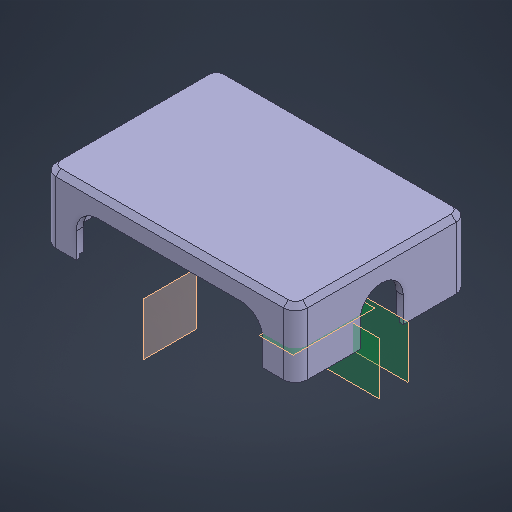
# Autodesk Inventor part: case2
Saved by Autodesk Inventor 2025.2 (Build 292293000, 293)
## iProperties
Created: 2025-10-05
Part Number: case2
Material: Generic
Document SubType Name: Modeling
Designer: micyg
Density: 1 g/cm^3
Appearance: Default
Sheet Metal Rule: Default
Author: micyg
## iProperties of the stored document case2_3DPrint.ipt
Created: 2025-10-05
Part Number: case2_3DPrint
Material: Generic
Document SubType Name: Modeling
Designer: micyg
Density: 1 g/cm^3
Appearance: Default
Author: micyg
Autodesk Inventor part; units mm, degrees
ref_plane "YZ Plane" through (0, 0, 0) normal (1, 0, 0) x (0, 1, 0)
ref_plane "XZ Plane" through (0, 0, 0) normal (0, 1, 0) x (-1, 0, 0)
ref_plane "XY Plane" through (0, 0, 0) normal (0, 0, 1) x (1, 0, 0)
sketch "Sketch1" plane through (0, 0, 0) normal (0, 1, 0) x (-1, 0, 0)
  line L0 (0, 0) -> (105.2, 0)
  line L1 (105.2, 0) -> (105.2, -72.2)
  line L2 (105.2, -72.2) -> (0, -72.2)
  line L3 (0, -72.2) -> (0, 0)
  dimension "d0" = 105.2
  dimension "d1" = 72.2
  constraints: 8 end point, 2 parallel, 1 horizontal, 1 perpendicular
  measures "d0" distance of L1.end L2.end
  measures "d1" distance of L0.end L1.end
extrude "Extrusion1" add sketch "Sketch1" along normal blind 28
fillet "Fillet1" radius 5 4 edges at (-105.2, 14, 0) (0, 14, 0) (-105.2, 14, -72.2) (0, 14, -72.2)
chamfer "Chamfer1" distance 2 angle 45 8 edges at (-52.6, 28, 0) (-1.4645, 28, -1.4645) (0, 28, -36.1) (-1.4645, 28, -70.7355) (-52.6, 28, -72.2) (-103.7355, 28, -70.7355) (-105.2, 28, -36.1) (-103.7355, 28, -1.4645)
shell "Shell2" thickness 3 removed faces 1 at (-36.7333, 0, -24.0667)
sketch "Sketch2" plane through (0, 0, 0) normal (0, -1, 0) x (1, 0, 0)
  arc A0 (-5, -69.2) -> (-3, -67.2) centre (-5, -67.2) ccw projected
  line L0 (-5, -69.2) -> (-100.2, -69.2) projected
  arc A1 (-102.2, -67.2) -> (-100.2, -69.2) centre (-100.2, -67.2) ccw projected
  line L1 (-102.2, -67.2) -> (-102.2, -5) projected
  arc A2 (-100.2, -3) -> (-102.2, -5) centre (-100.2, -5) ccw projected
  line L2 (-100.2, -3) -> (-5, -3) projected
  arc A3 (-3, -5) -> (-5, -3) centre (-5, -5) ccw projected
  line L3 (-3, -5) -> (-3, -67.2) projected
  arc A4 (-5, -72.2) -> (0, -67.2) centre (-5, -67.2) ccw projected
  line L4 (0, -5) -> (0, -67.2) projected
  arc A5 (0, -5) -> (-5, 0) centre (-5, -5) ccw projected
  line L5 (-100.2, 0) -> (-5, 0) projected
  arc A6 (-100.2, 0) -> (-105.2, -5) centre (-100.2, -5) ccw projected
  line L6 (-105.2, -67.2) -> (-105.2, -5) projected
  arc A7 (-105.2, -67.2) -> (-100.2, -72.2) centre (-100.2, -67.2) ccw projected
  line L7 (-5, -72.2) -> (-100.2, -72.2) projected
  arc A8 (-5, -70.8) -> (-1.4, -67.2) centre (-5, -67.2) ccw
  line L8 (-5, -70.8) -> (-100.2, -70.8)
  arc A9 (-103.8, -67.2) -> (-100.2, -70.8) centre (-100.2, -67.2) ccw
  line L9 (-103.8, -67.2) -> (-103.8, -5)
  arc A10 (-100.2, -1.4) -> (-103.8, -5) centre (-100.2, -5) ccw
  line L10 (-100.2, -1.4) -> (-5, -1.4)
  arc A11 (-1.4, -5) -> (-5, -1.4) centre (-5, -5) ccw
  line L11 (-1.4, -5) -> (-1.4, -67.2)
  point P0 (0, 0)
  dimension "d8" = 1.4
  constraints: 8 end point, 8 point on circle, 4 centre point, 7 other
  measures "d8" distance between parallel lines of L4 L11
extrude "Extrusion2" cut sketch "Sketch2" against normal blind 1.6 contours L8 A9 L9 A10 L10 A11 L11 A8
ref_plane "Work Plane2" through (-52.6, 0, 0) normal (1, 0, 0) x (0, 1, 0)
ref_plane "Work Plane3" through (0, 0, -36.1) normal (0, 0, -1) x (-1, 0, 0)
ref_plane "Work Plane4" through (0, 12.5, 0) normal (0, -1, 0) x (1, 0, 0)
sketch "Sketch19" plane through (-52.6, 0, 0) normal (1, 0, 0) x (0, 1, 0)
  line L0 (1.6, -3) -> (24.7574, -3) projected
  line L1 (24.7574, -3) -> (1.6, -3) projected
  arc A0 (25, -4) -> (24, -3) centre (24, -4) ccw projected
  arc A1 (25, -4) -> (24, -3) centre (24, -4) ccw projected
  line L2 (25, -68.2) -> (25, -67.2) projected
  line L3 (25, -67.2) -> (25, -5) projected
  line L4 (25, -5) -> (25, -4) projected
  line L5 (25, -4) -> (25, -5) projected
  line L6 (25, -5) -> (25, -67.2) projected
  line L7 (25, -67.2) -> (25, -68.2) projected
  line L8 (25, -5.7) -> (18, -5.7)
  line L9 (17, -5.7) -> (18, -6.7) construction
  line L10 (18, -6.7) -> (18, -5.7)
  line L11 (18, -5.7) -> (17, -5.7) construction
  line L12 (18, -6.7) -> (25, -13.7)
  line L13 (0, -67.2) -> (0, -70.8) projected
  line L14 (0, -70.8) -> (0, -67.2) projected
  line L15 (0, -67.2) -> (0, -5) projected
  line L16 (0, -5) -> (0, -1.4) projected
  line L17 (0, -1.4) -> (0, -5) projected
  line L18 (0, -5) -> (0, -67.2) projected
  line L19 (0, -67.2) -> (0, -72.2) projected
  line L20 (0, -5) -> (0, -67.2) projected
  line L21 (0, 0) -> (0, -5) projected
  line L22 (0, -5) -> (0, 0) projected
  line L23 (0, -67.2) -> (0, -5) projected
  line L24 (0, -72.2) -> (0, -67.2) projected
  dimension "d103" = 45
  dimension "d104" = 2.7
  dimension "d105" = 1
  dimension "d106" = 18
  constraints: 10 end point, 4 perpendicular, 2 point on line, 1 collinear
  measures "d103" angle of L3 L9
  measures "d104" distance between parallel lines of L0 L8
  measures "d105" distance from line of L9.end L8
  measures "d106" distance between parallel lines of L15 L10
extrude "Extrusion15" add sketch "Sketch19" against normal up to surface (49.6 mm away)
mirror "Mirror9" about plane through (-52.6, 0, 0) normal (1, 0, 0) of "Extrusion15"
mirror "Mirror10" about plane through (0, 0, -36.1) normal (0, 0, -1) of "Extrusion15", "Mirror9"
sketch "Sketch9" plane through (0, 12.5, 0) normal (0, -1, 0) x (1, 0, 0)
  arc A0 (-5, -70.8) -> (-1.4, -67.2) centre (-5, -67.2) ccw projected
  line L0 (-5, -70.8) -> (-100.2, -70.8) projected
  arc A1 (-103.8, -67.2) -> (-100.2, -70.8) centre (-100.2, -67.2) ccw projected
  line L1 (-103.8, -67.2) -> (-103.8, -5) projected
  arc A2 (-100.2, -1.4) -> (-103.8, -5) centre (-100.2, -5) ccw projected
  line L2 (-100.2, -1.4) -> (-5, -1.4) projected
  arc A3 (-1.4, -5) -> (-5, -1.4) centre (-5, -5) ccw projected
  line L3 (-1.4, -5) -> (-1.4, -67.2) projected
  arc A4 (-5, -72.2) -> (0, -67.2) centre (-5, -67.2) ccw projected
  line L4 (0, -5) -> (0, -67.2) projected
  arc A5 (0, -5) -> (-5, 0) centre (-5, -5) ccw projected
  line L5 (-100.2, 0) -> (-5, 0) projected
  arc A6 (-100.2, 0) -> (-105.2, -5) centre (-100.2, -5) ccw projected
  line L6 (-105.2, -67.2) -> (-105.2, -5) projected
  arc A7 (-105.2, -67.2) -> (-100.2, -72.2) centre (-100.2, -67.2) ccw projected
  line L7 (-5, -72.2) -> (-100.2, -72.2) projected
  line L8 (-5, -70.8) -> (-100.2, -70.8) projected
  arc A8 (-5, -70.8) -> (-1.4, -67.2) centre (-5, -67.2) ccw projected
  line L9 (-1.4, -5) -> (-1.4, -67.2) projected
  arc A9 (-1.4, -5) -> (-5, -1.4) centre (-5, -5) ccw projected
  line L10 (-100.2, -1.4) -> (-5, -1.4) projected
  arc A10 (-100.2, -1.4) -> (-103.8, -5) centre (-100.2, -5) ccw projected
  line L11 (-103.8, -67.2) -> (-103.8, -5) projected
  arc A11 (-103.8, -67.2) -> (-100.2, -70.8) centre (-100.2, -67.2) ccw projected
  line L12 (-102.2, -5) -> (-102.2, -67.2) projected
  arc A12 (-100.2, -3) -> (-102.2, -5) centre (-100.2, -5) ccw projected
  line L13 (-5, -3) -> (-100.2, -3) projected
  arc A13 (-3, -5) -> (-5, -3) centre (-5, -5) ccw projected
  line L14 (-3, -67.2) -> (-3, -5) projected
  arc A14 (-5, -69.2) -> (-3, -67.2) centre (-5, -67.2) ccw projected
  line L15 (-100.2, -69.2) -> (-5, -69.2) projected
  arc A15 (-102.2, -67.2) -> (-100.2, -69.2) centre (-100.2, -67.2) ccw projected
  line L16 (-96.7, -8.6) -> (-8.7, -8.6) construction
  line L17 (-8.7, -8.6) -> (-8.7, -63.6) construction
  line L18 (-8.7, -63.6) -> (-96.7, -63.6) construction
  line L19 (-96.7, -63.6) -> (-96.7, -8.6) construction
  circle A16 centre (-96.7, -8.6) radius 1.5
  circle A17 centre (-8.7, -8.6) radius 1.5
  circle A18 centre (-96.7, -63.6) radius 1.5
  circle A19 centre (-8.7, -63.6) radius 1.5
  line L20 (-52.7, -8.6) -> (-52.7, -63.6) construction
  line L21 (-101.7, -3.6) -> (-3.7, -3.6) construction
  line L22 (-3.7, -3.6) -> (-3.7, -68.6) construction
  line L23 (-3.7, -68.6) -> (-101.7, -68.6) construction
  line L24 (-101.7, -68.6) -> (-101.7, -3.6) construction
  line L25 (-101.7, -36.1) -> (-3.7, -36.1) construction
  line L26 (-52.6, 0) -> (-52.6, -72.2) construction
  line L27 (-105.2, -36.1) -> (0, -36.1) construction
  line L28 (-93.2, -3) -> (-93.2, -8.6)
  line L29 (-102.2, -12.1) -> (-102.2, -5)
  arc A20 (-96.7, -12.1) -> (-93.2, -8.6) centre (-96.7, -8.6) ccw
  line L30 (-96.7, -12.1) -> (-102.2, -12.1)
  line L31 (-100.2, -3) -> (-93.2, -3)
  line L32 (-93.2, -69.2) -> (-93.2, -63.6)
  arc A21 (-93.2, -63.6) -> (-96.7, -60.1) centre (-96.7, -63.6) ccw
  line L33 (-96.7, -60.1) -> (-102.2, -60.1)
  arc A22 (-12.2, -8.6) -> (-8.7, -12.1) centre (-8.7, -8.6) ccw
  line L34 (-3, -12.1) -> (-3, -5)
  line L35 (-12.2, -3) -> (-12.2, -8.6)
  line L36 (-8.7, -12.1) -> (-3, -12.1)
  line L37 (-5, -3) -> (-12.2, -3)
  arc A23 (-8.7, -60.1) -> (-12.2, -63.6) centre (-8.7, -63.6) ccw
  line L38 (-12.2, -69.2) -> (-12.2, -63.6)
  line L39 (-8.7, -60.1) -> (-3, -60.1)
  line L40 (-93.2, -3) -> (-95.2, -3)
  line L41 (-95.2, -3) -> (-95.2, -6)
  line L42 (-95.2, -6) -> (-93.2, -6)
  line L43 (-93.2, -6) -> (-93.2, -3)
  line L44 (-12.2, -3) -> (-10.2, -3)
  line L45 (-10.2, -3) -> (-10.2, -6)
  line L46 (-10.2, -6) -> (-12.2, -6)
  line L47 (-12.2, -6) -> (-12.2, -3)
  line L48 (-95.2, -69.2) -> (-95.2, -66.2)
  line L49 (-95.2, -66.2) -> (-93.2, -66.2)
  line L50 (-10.2, -69.2) -> (-10.2, -66.2)
  line L51 (-10.2, -66.2) -> (-12.2, -66.2)
  arc A24 (-3, -5) -> (-5, -3) centre (-5, -5) ccw projected
  line L52 (-5, -3) -> (-100.2, -3) projected
  arc A25 (-100.2, -3) -> (-102.2, -5) centre (-100.2, -5) ccw projected
  line L53 (-102.2, -5) -> (-102.2, -67.2) projected
  arc A26 (-102.2, -67.2) -> (-100.2, -69.2) centre (-100.2, -67.2) ccw projected
  line L54 (-100.2, -69.2) -> (-5, -69.2) projected
  arc A27 (-5, -69.2) -> (-3, -67.2) centre (-5, -67.2) ccw projected
  line L55 (-3, -67.2) -> (-3, -5) projected
  arc A28 (0, -5) -> (-5, 0) centre (-5, -5) ccw projected
  line L56 (0, -5) -> (0, -67.2) projected
  arc A29 (-5, -72.2) -> (0, -67.2) centre (-5, -67.2) ccw projected
  line L57 (-5, -72.2) -> (-100.2, -72.2) projected
  arc A30 (-105.2, -67.2) -> (-100.2, -72.2) centre (-100.2, -67.2) ccw projected
  line L58 (-105.2, -67.2) -> (-105.2, -5) projected
  arc A31 (-100.2, 0) -> (-105.2, -5) centre (-100.2, -5) ccw projected
  line L59 (-100.2, 0) -> (-5, 0) projected
  arc A32 (-3, -5) -> (-5, -3) centre (-5, -5) ccw projected
  line L60 (-5, -3) -> (-100.2, -3) projected
  arc A33 (-100.2, -3) -> (-102.2, -5) centre (-100.2, -5) ccw projected
  line L61 (-102.2, -5) -> (-102.2, -67.2) projected
  arc A34 (-102.2, -67.2) -> (-100.2, -69.2) centre (-100.2, -67.2) ccw projected
  line L62 (-100.2, -69.2) -> (-5, -69.2) projected
  arc A35 (-5, -69.2) -> (-3, -67.2) centre (-5, -67.2) ccw projected
  line L63 (-3, -67.2) -> (-3, -5) projected
  arc A36 (0, -5) -> (-5, 0) centre (-5, -5) ccw projected
  line L64 (0, -5) -> (0, -67.2) projected
  arc A37 (-5, -72.2) -> (0, -67.2) centre (-5, -67.2) ccw projected
  line L65 (-5, -72.2) -> (-100.2, -72.2) projected
  arc A38 (-105.2, -67.2) -> (-100.2, -72.2) centre (-100.2, -67.2) ccw projected
  line L66 (-105.2, -67.2) -> (-105.2, -5) projected
  arc A39 (-100.2, 0) -> (-105.2, -5) centre (-100.2, -5) ccw projected
  line L67 (-100.2, 0) -> (-5, 0) projected
  point P0 (-52.7, -36.1)
  dimension "d137" = 88
  dimension "d138" = 55
  dimension "d139" = 3
  dimension "d140" = 3
  dimension "d141" = 3
  dimension "d142" = 3
  dimension "d143" = 98
  dimension "d144" = 65
  dimension "d145" = 0.5
  dimension "d147" = 2
  dimension "d148" = 2
  dimension "d149" = 3
  dimension "d150" = 2
  constraints: 72 end point, 16 symmetric about line, 12 parallel, 12 point on circle, 10 midpoint, 8 centre point, 6 horizontal, 6 perpendicular, 6 point on line, 5 coincident, 4 tangent, 1 collinear, 3 other
  measures "d137" distance of L16.start L16.end
  measures "d138" distance of L18.end L16.start
  measures "d139" diameter of A16
  measures "d140" diameter of A19
  measures "d141" diameter of A17
  measures "d142" diameter of A18
  measures "d143" distance of L21.start L21.end
  measures "d144" distance of L23.end L21.start
  measures "d145" distance between parallel lines of L12 L24
  measures "d147" radial gap between concentric circles of A16 A20
  measures "d148" radial gap between concentric circles of A22 A17
  measures "d149" distance between parallel lines of L13 L42
  measures "d150" distance between parallel lines of L28 L41
extrude "Extrusion13" add sketch "Sketch9" against normal up to surface (12.5 mm away) contours A12 L13 L41 L42 L28 A20 L30 L12 | L33 A21 L32 L49 L48 L15 A15 L12 | L13 A13 L14 L36 A22 L35 L46 L45 | L50 L51 L38 A23 L39 L14 A14 L15 | A16 | A17 | A18 | A19
sketch "Sketch18" plane through (-105.2, 0, -67.2) normal (-1, 0, 0) x (0, 0, 1)
  line L0 (26.03, 2.015) -> (26.03, 2.615)
  arc A0 (27.81, 4.395) -> (26.03, 2.615) centre (27.81, 2.615) ccw
  arc A1 (26.03, 2.015) -> (27.81, 0.235) centre (27.81, 2.015) ccw construction
  line L1 (27.81, 0.235) -> (31.1061, 0.235)
  line L2 (34.19, 0.235) -> (31.1061, 0.235)
  arc A2 (34.19, 0.235) -> (35.97, 2.015) centre (34.19, 2.015) ccw construction
  line L3 (35.97, 2.615) -> (35.97, 2.015)
  arc A3 (35.97, 2.615) -> (34.19, 4.395) centre (34.19, 2.615) ccw
  line L4 (27.81, 4.395) -> (34.19, 4.395)
  line L5 (35.97, 2.015) -> (26.03, 2.015) construction
  line L6 (26.03, 2.015) -> (26.03, 0.235)
  line L7 (35.97, 0.235) -> (35.97, 2.015)
  line L8 (31, 0.935) -> (31, 0.735) projected
  line L9 (27.81, 0.935) -> (31, 0.935) projected
  arc A4 (26.73, 2.015) -> (27.81, 0.935) centre (27.81, 2.015) ccw projected
  line L10 (26.73, 2.615) -> (26.73, 2.015) projected
  arc A5 (27.81, 3.695) -> (26.73, 2.615) centre (27.81, 2.615) ccw projected
  line L11 (31, 3.695) -> (27.81, 3.695) projected
  line L12 (31, 3.895) -> (31, 3.695) projected
  line L13 (31, 3.895) -> (27.81, 3.895) projected
  arc A6 (27.81, 3.895) -> (26.53, 2.615) centre (27.81, 2.615) ccw projected
  line L14 (26.53, 2.615) -> (26.53, 2.015) projected
  arc A7 (26.53, 2.015) -> (27.81, 0.735) centre (27.81, 2.015) ccw projected
  line L15 (27.81, 0.735) -> (31, 0.735) projected
  line L16 (31, 0.935) -> (31, 0.735) projected
  line L17 (34.19, 0.735) -> (31, 0.735) projected
  arc A8 (34.19, 0.735) -> (35.47, 2.015) centre (34.19, 2.015) ccw projected
  line L18 (35.47, 2.615) -> (35.47, 2.015) projected
  arc A9 (35.47, 2.615) -> (34.19, 3.895) centre (34.19, 2.615) ccw projected
  line L19 (31, 3.895) -> (34.19, 3.895) projected
  line L20 (31, 3.895) -> (31, 3.695) projected
  line L21 (31, 3.695) -> (34.19, 3.695) projected
  arc A10 (35.27, 2.615) -> (34.19, 3.695) centre (34.19, 2.615) ccw projected
  line L22 (35.27, 2.615) -> (35.27, 2.015) projected
  arc A11 (34.19, 0.935) -> (35.27, 2.015) centre (34.19, 2.015) ccw projected
  line L23 (34.19, 0.935) -> (31, 0.935) projected
  line L24 (26.03, 0.235) -> (35.97, 0.235)
  line L25 (0, 0) -> (0, 26) projected
  line L26 (0, 0) -> (62.2, 0) projected
  line L27 (62.2, 26) -> (62.2, 0) projected
  line L28 (0, 0) -> (62.2, 0) projected
  line L29 (35.97, 0.235) -> (26.03, 0.235)
  line L30 (26.03, 0.235) -> (26.03, 0)
  line L31 (26.03, 0) -> (35.97, 0)
  line L32 (35.97, 0) -> (35.97, 0.235)
  line L33 (0, 26) -> (62.2, 26) projected
  point P0 (67.2, 0)
  dimension "d136" = 0.5
  constraints: 26 end point, 8 point on circle, 8 tangent, 4 centre point, 4 coincident, 4 horizontal, 3 parallel, 2 perpendicular, 2 point on line, 1 collinear
  measures "d136" distance between parallel lines of L4 L13
extrude "Extrusion14" cut sketch "Sketch18" against normal up to surface (3 mm away) contours L0 A0 L4 A3 L3 L7 L24 L2 L1 L6 | L24 L1 L2 L32 L26 L30 | L23 A11 L22 A10 L21 L12 L19 A9 L18 A8 L17 L8 | L8 L15 A7 L14 A6 L13 L12 L11 A5 L10 A4 L9 | L9 A4 L10 A5 L11 L21 A10 L22 A11 L23
sketch "Sketch20" plane through (0, 0, -5) normal (1, 0, 0) x (0, 0, -1)
  circle A0 centre (31.1, 10.585) radius 9
  line L0 (40.1, 10.585) -> (22.1, 10.585) construction
  line L1 (22.1, 10.585) -> (22.1, 0)
  line L2 (22.1, 0) -> (40.1, 0)
  line L3 (40.1, 0) -> (40.1, 10.585)
  line L4 (0, 0) -> (0, 26) construction
  line L5 (0, 0) -> (62.2, 0) construction
  line L6 (62.2, 26) -> (62.2, 0) construction
  line L7 (0, 0) -> (62.2, 0) construction
  circle A1 centre (31.1, 10.585) radius 7 construction
  line L8 (0, 26) -> (62.2, 26) projected
  point P0 (-5, 0)
  dimension "d109" = 18
  constraints: 8 end point, 2 parallel, 2 point on circle, 1 centre point, 1 coincident, 1 horizontal, 1 midpoint, 1 perpendicular, 1 point on line, 1 tangent
  measures "d109" diameter of A0
extrude "Extrusion16" cut sketch "Sketch20" against normal up to surface (3 mm away)
sketch "Sketch21" plane through (-5, 0, -72.2) normal (0, 0, -1) x (-1, 0, 0)
  line L0 (87.5, 0.585) -> (67.5, 0.585) construction
  line L1 (87.5, 0.585) -> (87.5, 20.085) construction
  line L2 (67.5, 20.085) -> (87.5, 20.085) construction
  line L3 (67.5, 20.085) -> (67.5, 0.585) construction
  line L4 (67.5, 0.585) -> (47.5, 0.585) construction
  line L5 (67.5, 0.585) -> (67.5, 20.085) construction
  line L6 (47.5, 20.085) -> (67.5, 20.085) construction
  line L7 (47.5, 20.085) -> (47.5, 0.585) construction
  line L8 (47.5, 0.585) -> (27.5, 0.585) construction
  line L9 (47.5, 0.585) -> (47.5, 20.085) construction
  line L10 (27.5, 20.085) -> (47.5, 20.085) construction
  line L11 (27.5, 20.085) -> (27.5, 0.585) construction
  line L12 (27.5, 0.585) -> (7.5, 0.585) construction
  line L13 (27.5, 0.585) -> (27.5, 20.085) construction
  line L14 (7.5, 20.085) -> (27.5, 20.085) construction
  line L15 (7.5, 20.085) -> (7.5, 0.585) construction
  circle A0 centre (17.7, 10.585) radius 9
  circle A1 centre (37.7, 10.585) radius 9
  circle A2 centre (57.7, 10.585) radius 9
  circle A3 centre (77.7, 10.585) radius 9
  line L16 (0, 0) -> (0, 26) construction
  line L17 (0, 0) -> (95.2, 0) projected
  line L18 (95.2, 26) -> (95.2, 0) construction
  line L19 (8.7, 10.585) -> (26.7, 10.585) construction
  line L20 (26.7, 10.585) -> (26.7, 0)
  line L21 (26.7, 0) -> (8.7, 0)
  line L22 (8.7, 0) -> (8.7, 10.585)
  line L23 (28.7, 10.585) -> (46.7, 10.585) construction
  line L24 (46.7, 10.585) -> (46.7, 0)
  line L25 (46.7, 0) -> (28.7, 0)
  line L26 (28.7, 0) -> (28.7, 10.585)
  line L27 (48.7, 10.585) -> (66.7, 10.585) construction
  line L28 (66.7, 10.585) -> (66.7, 0)
  line L29 (66.7, 0) -> (48.7, 0)
  line L30 (48.7, 0) -> (48.7, 10.585)
  line L31 (68.7, 10.585) -> (86.7, 10.585) construction
  line L32 (86.7, 10.585) -> (86.7, 0)
  line L33 (86.7, 0) -> (68.7, 0)
  line L34 (68.7, 0) -> (68.7, 10.585)
  line L35 (17.7, 19.585) -> (77.7, 19.585)
  circle A4 centre (17.7, 10.585) radius 7 projected
  circle A5 centre (37.7, 10.585) radius 7 projected
  circle A6 centre (57.7, 10.585) radius 7 projected
  circle A7 centre (77.7, 10.585) radius 7 projected
  line L36 (0, 26) -> (95.2, 26) projected
  point P0 (8.7, 0)
  dimension "d132" = 18
  dimension "d133" = 18
  dimension "d134" = 18
  dimension "d135" = 18
  constraints: 34 end point, 10 point on circle, 8 parallel, 6 point on line, 4 centre point, 4 horizontal, 4 perpendicular, 4 tangent, 3 coincident, 3 midpoint, 2 concentric
  measures "d132" diameter of A0
  measures "d133" diameter of A1
  measures "d134" diameter of A2
  measures "d135" diameter of A3
extrude "Extrusion17" cut sketch "Sketch21" against normal up to surface (3 mm away) contours A0 | L20 L17 L22 A0 | A0 L35 A1 L26 L17 L20 | L35 A2 L30 L17 L24 A1 | A1 | L26 A1 L24 L17 | L35 A3 L34 L17 L28 A2 | A2 | L28 L17 L30 A2 | A3 | L32 L17 L34 A3 | A4 | A5 | A6 | A7
mirror "Mirror11" about plane through (0, 0, -36.1) normal (0, 0, -1) of "Extrusion17"
ref_plane "Work Plane6" through (0, 0, -24.1) normal (0, 0, -1) x (-1, 0, 0)
sketch "Sketch22" plane through (0, 0, -24.1) normal (0, 0, -1) x (-1, 0, 0)
  line L0 (3, 10.585) -> (3, 1.6) projected
  line L1 (3, 1.6) -> (3, 12.5) projected
  line L2 (3, 12.5) -> (3, 1.6) projected
  line L3 (3, 1.6) -> (3, 10.585) projected
  line L4 (3, 10.585) -> (3, 10.585) projected
  arc A0 (4, 25) -> (3, 24) centre (4, 24) ccw projected
  arc A1 (4, 25) -> (3, 24) centre (4, 24) ccw projected
  line L5 (101.9574, 25) -> (3.2426, 25) projected
  line L6 (3.2426, 25) -> (101.9574, 25) projected
  arc A2 (102.2, 24) -> (101.2, 25) centre (101.2, 24) ccw projected
  arc A3 (102.2, 24) -> (101.2, 25) centre (101.2, 24) ccw projected
  line L7 (102.2, 2.615) -> (102.2, 1.6) projected
  line L8 (102.2, 1.6) -> (102.2, 12.5) projected
  line L9 (102.2, 12.5) -> (102.2, 1.6) projected
  line L10 (102.2, 1.6) -> (102.2, 2.615) projected
  line L11 (102.2, 2.615) -> (102.2, 4.395) projected
  line L12 (102.2, 4.395) -> (102.2, 2.615) projected
  line L13 (3, 5) -> (23, 25)
  line L14 (82.2, 25) -> (102.2, 5)
  line L15 (101.2, 25) -> (10.2, 25) projected
  line L16 (12.115, 25) -> (6.7, 19.585)
  line L17 (6.7, 19.585) -> (5.7, 19.585)
  line L18 (5.7, 19.585) -> (5.7, 25)
  line L19 (100.2, 0) -> (91.7, 0) projected
  line L20 (5, 26) -> (5, 0) projected
  line L21 (100.2, 0) -> (100.2, 26) projected
  line L22 (102.2, 23.4) -> (102.2, 24.7574) projected
  line L23 (3, 24.7574) -> (3, 23.4) projected
  line L24 (102.2, 24.7574) -> (102.2, 23.4) projected
  line L25 (3, 23.4) -> (3, 24.7574) projected
  line L26 (91.7, 0) -> (91.7, 10.585) construction
  arc A4 (91.7, 10.585) -> (82.7, 19.585) centre (82.7, 10.585) ccw construction
  line L27 (82.7, 19.585) -> (22.7, 19.585) construction
  arc A5 (22.7, 19.585) -> (13.7, 10.585) centre (22.7, 10.585) ccw construction
  line L28 (13.7, 10.585) -> (13.7, 0) construction
  line L29 (13.7, 0) -> (5, 0) projected
  line L30 (102.2, 12.5) -> (102.2, 23.4) projected
  line L31 (102.2, 23.4) -> (102.2, 12.5) projected
  line L32 (3, 12.5) -> (3, 23.4) projected
  line L33 (3, 23.4) -> (3, 12.5) projected
  line L34 (100.2, 26) -> (5, 26) projected
  point P0 (0, 0)
  point P1 (4, 25)
  point P2 (101.2, 25)
  point P3 (3, 5)
  point P4 (3, 10.585)
  point P5 (102.2, 5)
  point P6 (102.2, 24)
  point P7 (3, 18)
  dimension "d119" = 45
  dimension "d120" = 45
  dimension "d121" = 20
  dimension "d122" = 20
  dimension "d125" = 45
  dimension "d127" = 1
  dimension "d153" = 2.7
  constraints: 10 end point, 6 point on line, 1 collinear, 1 parallel, 1 perpendicular
  measures "d119" angle of L6 L14
  measures "d120" angle of L13 L6
  measures "d121" distance from line of L5 L13.start
  measures "d122" distance from line of L5 L14.end
  measures "d125" angle of L5 L16
  measures "d127" distance from line of L16.end L18
  measures "d153" distance between parallel lines of L32 L18
extrude "Extrusion18" add sketch "Sketch22" along normal mid plane 2 contours L5 L21 L14 | L5 A2 L22 L30 L8 L14 L21
mirror "Mirror12" about plane through (0, 0, -36.1) normal (0, 0, -1) of "Extrusion18"
extrude "Extrusion19" add sketch "Sketch22" along normal up to surface (23 mm away) contours L16 L17 L18 L5
sketch "Sketch26" plane through (0, 12.5, 0) normal (0, -1, 0) x (1, 0, 0)
  line L0 (-13.9061, -72.2) -> (-13.9061, -69.2) projected
  line L1 (-13.9061, -69.2) -> (-10.2, -69.2) projected
  line L2 (-5, -69.2) -> (-10.2, -69.2) projected
  arc A0 (-5, -69.2) -> (-3, -67.2) centre (-5, -67.2) ccw projected
  line L3 (-3, -67.2) -> (-3, -60.1) projected
  line L4 (-3, -60.1) -> (-3, -44.8939) projected
  line L5 (0, -27.3061) -> (-3, -27.3061) projected
  line L6 (0, -44.8939) -> (0, -67.2) projected
  arc A1 (-5, -72.2) -> (0, -67.2) centre (-5, -67.2) ccw projected
  line L7 (-5, -72.2) -> (-13.9061, -72.2) projected
  line L8 (-10.2, -69.2) -> (-10.2, -66.2) projected
  line L9 (-10.2, -66.2) -> (-12.2, -66.2) projected
  line L10 (-12.2, -66.2) -> (-12.2, -63.6) projected
  arc A2 (-8.7, -60.1) -> (-12.2, -63.6) centre (-8.7, -63.6) ccw projected
  line L11 (-8.7, -60.1) -> (-3, -60.1) projected
  line L12 (-10.2, -6) -> (-10.2, -3) projected
  line L13 (-10.2, -3) -> (-5, -3) projected
  arc A3 (-3, -5) -> (-5, -3) centre (-5, -5) ccw projected
  line L14 (-3, -12.1) -> (-3, -5) projected
  line L15 (-3, -27.3061) -> (-3, -12.1) projected
  line L16 (-3, -44.8939) -> (0, -44.8939) projected
  line L17 (0, -5) -> (0, -27.3061) projected
  arc A4 (0, -5) -> (-5, 0) centre (-5, -5) ccw projected
  line L18 (-13.9061, 0) -> (-5, 0) projected
  line L19 (-13.9061, -3) -> (-13.9061, 0) projected
  line L20 (-10.2, -3) -> (-13.9061, -3) projected
  line L21 (-12.2, -6) -> (-10.2, -6) projected
  line L22 (-12.2, -8.6) -> (-12.2, -6) projected
  arc A5 (-12.2, -8.6) -> (-8.7, -12.1) centre (-8.7, -8.6) ccw projected
  line L23 (-3, -12.1) -> (-8.7, -12.1) projected
  line L24 (-95.2, -3) -> (-95.2, -6) projected
  line L25 (-95.2, -6) -> (-93.2, -6) projected
  line L26 (-93.2, -6) -> (-93.2, -8.6) projected
  arc A6 (-96.7, -12.1) -> (-93.2, -8.6) centre (-96.7, -8.6) ccw projected
  line L27 (-96.7, -12.1) -> (-102.2, -12.1) projected
  line L28 (-102.2, -12.1) -> (-102.2, -5) projected
  arc A7 (-100.2, -3) -> (-102.2, -5) centre (-100.2, -5) ccw projected
  line L29 (-100.2, -3) -> (-95.2, -3) projected
  line L30 (-91.4939, -3) -> (-95.2, -3) projected
  line L31 (-91.4939, 0) -> (-91.4939, -3) projected
  line L32 (-100.2, 0) -> (-91.4939, 0) projected
  arc A8 (-100.2, 0) -> (-105.2, -5) centre (-100.2, -5) ccw projected
  line L33 (-105.2, -67.2) -> (-105.2, -5) projected
  arc A9 (-105.2, -67.2) -> (-100.2, -72.2) centre (-100.2, -67.2) ccw projected
  line L34 (-91.4939, -72.2) -> (-100.2, -72.2) projected
  line L35 (-91.4939, -69.2) -> (-91.4939, -72.2) projected
  line L36 (-95.2, -69.2) -> (-91.4939, -69.2) projected
  line L37 (-95.2, -69.2) -> (-100.2, -69.2) projected
  arc A10 (-102.2, -67.2) -> (-100.2, -69.2) centre (-100.2, -67.2) ccw projected
  line L38 (-102.2, -67.2) -> (-102.2, -60.1) projected
  line L39 (-102.2, -12.1) -> (-102.2, -23.1) projected
  line L40 (-95.2, -66.2) -> (-95.2, -69.2) projected
  line L41 (-93.2, -66.2) -> (-95.2, -66.2) projected
  line L42 (-93.2, -63.6) -> (-93.2, -66.2) projected
  arc A11 (-93.2, -63.6) -> (-96.7, -60.1) centre (-96.7, -63.6) ccw projected
  line L43 (-102.2, -60.1) -> (-96.7, -60.1) projected
  circle A12 centre (-96.7, -63.6) radius 1.5 projected
  circle A13 centre (-96.7, -8.6) radius 1.5 projected
  circle A14 centre (-8.7, -8.6) radius 1.5 projected
  circle A15 centre (-8.7, -63.6) radius 1.5 projected
  line L44 (-102.2, -23.1) -> (-94.7, -23.1) projected
  line L45 (-94.7, -23.1) -> (-94.7, -25.1) projected
  line L46 (-94.7, -25.1) -> (-102.2, -25.1) projected
  line L47 (-102.2, -25.1) -> (-102.2, -47.1) projected
  line L48 (-102.2, -47.1) -> (-94.7, -47.1) projected
  line L49 (-94.7, -47.1) -> (-94.7, -49.1) projected
  line L50 (-94.7, -49.1) -> (-102.2, -49.1) projected
  line L51 (-102.2, -49.1) -> (-102.2, -60.1) projected
  point P0 (0, 0)
extrude "Extrusion21" cut sketch "Sketch26" against normal up to surface (12.5 mm away) contours A12 | A13 | A14 | A15
equation "\"BendRadius\" = Thickness"
equation "\"BendReliefWidth\" = Thickness"
equation "\"BendReliefDepth\" = 0.5 * Thickness"
equation "\"CornerReliefSize\" = 4 * Thickness"
equation "\"MinimumRemnant\" = 2 * Thickness"
equation "\"TransitionRadius\" = BendRadius"
equation "\"JacobiRadiusSize\" = BendRadius"
equation "\"GapSize\" = Thickness"
equation "\"Thickness\" = 3.048"
body "Solid1"
